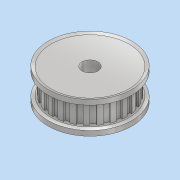
# Autodesk Inventor part: Koło zębate 21 T5 24 2F
Saved by Autodesk Inventor 2018 (Build 220112000, 112)
## iProperties
Created: 2019-01-23
Part Number: Koło zębate 21 T5 24 2F
Material: Ogólny
Document SubType Name: Modeling
Designer: Dawid
Density: 1 g/cm^3
Appearance: Aluminium — ciemne
Author: Dawid
Autodesk Inventor part; units mm, degrees
ref_plane "YZ Plane" through (0, 0, 0) normal (1, 0, 0) x (0, 1, 0)
ref_plane "XZ Plane" through (0, 0, 0) normal (0, 1, 0) x (-1, 0, 0)
ref_plane "XY Plane" through (0, 0, 0) normal (0, 0, 1) x (1, 0, 0)
sketch "Szkic1" plane through (0, 0, 0) normal (0, 0, 1) x (1, 0, 0)
  arc A0 (2.4408, 18.54) -> (0, 18.7) centre (0, 0) ccw
  arc A1 (0, 17.7) -> (2.3103, 17.5486) centre (0, 0) ccw
  line L0 (0, 0) -> (0, 18.7)
  line L1 (0, 0) -> (2.4408, 18.54)
  line L2 (0, 0) -> (18.7, 0) construction
  dimension "d0" = 37.4
  dimension "d1" = 35.4
  dimension "d2" = 82.5
  constraints: 6 end point, 4 point on circle, 2 centre point, 2 coincident, 2 point on line, 1 equal length, 1 horizontal, 1 vertical
  measures "d0" diameter of A0
  measures "d1" diameter of A1
  measures "d2" angle of L2 L1
extrude "Wyciągnięcie proste1" add sketch "Szkic1" along normal blind 21
pattern_circular "Szyk kołowy1" count 24 over 360 about axis through (0, 0, 0) along (0, 0, 1) of "Wyciągnięcie proste1"
sketch "Szkic2" plane through (0, 0, 0) normal (0, 0, -1) x (-1, 0, 0)
  line L0 (0, 18.7) -> (0, 17.7) projected
  arc A0 (0, 18.7) -> (-2.4408, 18.54) centre (0, 0) ccw projected
  line L1 (-2.3103, 17.5486) -> (-2.4408, 18.54) projected
  arc A1 (-2.3103, 17.5486) -> (-4.5811, 17.0969) centre (0, 0) ccw projected
  line L2 (-4.8399, 18.0628) -> (-4.5811, 17.0969) projected
  arc A2 (-4.8399, 18.0628) -> (-7.1562, 17.2765) centre (0, 0) ccw projected
  line L3 (-6.7735, 16.3527) -> (-7.1562, 17.2765) projected
  arc A3 (-6.7735, 16.3527) -> (-8.85, 15.3286) centre (0, 0) ccw projected
  line L4 (-9.35, 16.1947) -> (-8.85, 15.3286) projected
  arc A4 (-9.35, 16.1947) -> (-11.3838, 14.8357) centre (0, 0) ccw projected
  line L5 (-10.7751, 14.0424) -> (-11.3838, 14.8357) projected
  arc A5 (-10.7751, 14.0424) -> (-12.5158, 12.5158) centre (0, 0) ccw projected
  line L6 (-13.2229, 13.2229) -> (-12.5158, 12.5158) projected
  arc A6 (-13.2229, 13.2229) -> (-14.8357, 11.3838) centre (0, 0) ccw projected
  line L7 (-14.0424, 10.7751) -> (-14.8357, 11.3838) projected
  arc A7 (-14.0424, 10.7751) -> (-15.3286, 8.85) centre (0, 0) ccw projected
  line L8 (-16.1947, 9.35) -> (-15.3286, 8.85) projected
  arc A8 (-16.1947, 9.35) -> (-17.2765, 7.1562) centre (0, 0) ccw projected
  line L9 (-16.3527, 6.7735) -> (-17.2765, 7.1562) projected
  arc A9 (-16.3527, 6.7735) -> (-17.0969, 4.5811) centre (0, 0) ccw projected
  line L10 (-18.0628, 4.8399) -> (-17.0969, 4.5811) projected
  arc A10 (-18.0628, 4.8399) -> (-18.54, 2.4408) centre (0, 0) ccw projected
  line L11 (-17.5486, 2.3103) -> (-18.54, 2.4408) projected
  arc A11 (-17.5486, 2.3103) -> (-17.7, 0) centre (0, 0) ccw projected
  line L12 (-18.7, 0) -> (-17.7, 0) projected
  arc A12 (-18.7, 0) -> (-18.54, -2.4408) centre (0, 0) ccw projected
  line L13 (-17.5486, -2.3103) -> (-18.54, -2.4408) projected
  arc A13 (-17.5486, -2.3103) -> (-17.0969, -4.5811) centre (0, 0) ccw projected
  line L14 (-18.0628, -4.8399) -> (-17.0969, -4.5811) projected
  arc A14 (-18.0628, -4.8399) -> (-17.2765, -7.1562) centre (0, 0) ccw projected
  line L15 (-16.3527, -6.7735) -> (-17.2765, -7.1562) projected
  arc A15 (-16.3527, -6.7735) -> (-15.3286, -8.85) centre (0, 0) ccw projected
  line L16 (-16.1947, -9.35) -> (-15.3286, -8.85) projected
  arc A16 (-16.1947, -9.35) -> (-14.8357, -11.3838) centre (0, 0) ccw projected
  line L17 (-14.0424, -10.7751) -> (-14.8357, -11.3838) projected
  arc A17 (-14.0424, -10.7751) -> (-12.5158, -12.5158) centre (0, 0) ccw projected
  line L18 (-13.2229, -13.2229) -> (-12.5158, -12.5158) projected
  arc A18 (-13.2229, -13.2229) -> (-11.3838, -14.8357) centre (0, 0) ccw projected
  line L19 (-10.7751, -14.0424) -> (-11.3838, -14.8357) projected
  arc A19 (-10.7751, -14.0424) -> (-8.85, -15.3286) centre (0, 0) ccw projected
  line L20 (-9.35, -16.1947) -> (-8.85, -15.3286) projected
  arc A20 (-9.35, -16.1947) -> (-7.1562, -17.2765) centre (0, 0) ccw projected
  line L21 (-6.7735, -16.3527) -> (-7.1562, -17.2765) projected
  arc A21 (-6.7735, -16.3527) -> (-4.5811, -17.0969) centre (0, 0) ccw projected
  line L22 (-4.8399, -18.0628) -> (-4.5811, -17.0969) projected
  arc A22 (-4.8399, -18.0628) -> (-2.4408, -18.54) centre (0, 0) ccw projected
  line L23 (-2.3103, -17.5486) -> (-2.4408, -18.54) projected
  arc A23 (-2.3103, -17.5486) -> (0, -17.7) centre (0, 0) ccw projected
  line L24 (0, -18.7) -> (0, -17.7) projected
  arc A24 (0, -18.7) -> (2.4408, -18.54) centre (0, 0) ccw projected
  line L25 (2.3103, -17.5486) -> (2.4408, -18.54) projected
  arc A25 (2.3103, -17.5486) -> (4.5811, -17.0969) centre (0, 0) ccw projected
  line L26 (4.8399, -18.0628) -> (4.5811, -17.0969) projected
  arc A26 (4.8399, -18.0628) -> (7.1562, -17.2765) centre (0, 0) ccw projected
  line L27 (6.7735, -16.3527) -> (7.1562, -17.2765) projected
  arc A27 (6.7735, -16.3527) -> (8.85, -15.3286) centre (0, 0) ccw projected
  line L28 (9.35, -16.1947) -> (8.85, -15.3286) projected
  arc A28 (9.35, -16.1947) -> (11.3838, -14.8357) centre (0, 0) ccw projected
  line L29 (10.7751, -14.0424) -> (11.3838, -14.8357) projected
  arc A29 (10.7751, -14.0424) -> (12.5158, -12.5158) centre (0, 0) ccw projected
  line L30 (13.2229, -13.2229) -> (12.5158, -12.5158) projected
  arc A30 (13.2229, -13.2229) -> (14.8357, -11.3838) centre (0, 0) ccw projected
  line L31 (14.0424, -10.7751) -> (14.8357, -11.3838) projected
  arc A31 (14.0424, -10.7751) -> (15.3286, -8.85) centre (0, 0) ccw projected
  line L32 (16.1947, -9.35) -> (15.3286, -8.85) projected
  arc A32 (16.1947, -9.35) -> (17.2765, -7.1562) centre (0, 0) ccw projected
  line L33 (16.3527, -6.7735) -> (17.2765, -7.1562) projected
  arc A33 (16.3527, -6.7735) -> (17.0969, -4.5811) centre (0, 0) ccw projected
  line L34 (18.0628, -4.8399) -> (17.0969, -4.5811) projected
  arc A34 (18.0628, -4.8399) -> (18.54, -2.4408) centre (0, 0) ccw projected
  line L35 (17.5486, -2.3103) -> (18.54, -2.4408) projected
  arc A35 (17.5486, -2.3103) -> (17.7, 0) centre (0, 0) ccw projected
  line L36 (18.7, 0) -> (17.7, 0) projected
  arc A36 (18.7, 0) -> (18.54, 2.4408) centre (0, 0) ccw projected
  line L37 (17.5486, 2.3103) -> (18.54, 2.4408) projected
  arc A37 (17.5486, 2.3103) -> (17.0969, 4.5811) centre (0, 0) ccw projected
  line L38 (18.0628, 4.8399) -> (17.0969, 4.5811) projected
  arc A38 (18.0628, 4.8399) -> (17.2765, 7.1562) centre (0, 0) ccw projected
  line L39 (16.3527, 6.7735) -> (17.2765, 7.1562) projected
  arc A39 (16.3527, 6.7735) -> (15.3286, 8.85) centre (0, 0) ccw projected
  line L40 (16.1947, 9.35) -> (15.3286, 8.85) projected
  arc A40 (16.1947, 9.35) -> (14.8357, 11.3838) centre (0, 0) ccw projected
  line L41 (14.0424, 10.7751) -> (14.8357, 11.3838) projected
  arc A41 (14.0424, 10.7751) -> (12.5158, 12.5158) centre (0, 0) ccw projected
  line L42 (13.2229, 13.2229) -> (12.5158, 12.5158) projected
  arc A42 (13.2229, 13.2229) -> (11.3838, 14.8357) centre (0, 0) ccw projected
  line L43 (10.7751, 14.0424) -> (11.3838, 14.8357) projected
  arc A43 (10.7751, 14.0424) -> (8.85, 15.3286) centre (0, 0) ccw projected
  line L44 (9.35, 16.1947) -> (8.85, 15.3286) projected
  arc A44 (9.35, 16.1947) -> (7.1562, 17.2765) centre (0, 0) ccw projected
  line L45 (6.7735, 16.3527) -> (7.1562, 17.2765) projected
  arc A45 (6.7735, 16.3527) -> (4.5811, 17.0969) centre (0, 0) ccw projected
  line L46 (4.8399, 18.0628) -> (4.5811, 17.0969) projected
  arc A46 (4.8399, 18.0628) -> (2.4408, 18.54) centre (0, 0) ccw projected
  line L47 (2.3103, 17.5486) -> (2.4408, 18.54) projected
  arc A47 (2.3103, 17.5486) -> (0, 17.7) centre (0, 0) ccw projected
  circle A48 centre (0, 0) radius 12
  dimension "d8" = 24
  constraints: 1 centre point, 1 coincident
  measures "d8" diameter of A48
extrude "Wyciągnięcie proste2" cut sketch "Szkic2" against normal blind 6
sketch "Szkic3" plane through (0, 0, 0) normal (1, 0, 0) x (0, 1, 0)
  line L0 (0, 6) -> (-2.3103, 6) projected
  line L1 (0, 6) -> (19.5, 6)
  line L2 (21, 6) -> (21, 5.5)
  line L3 (19.5, 6) -> (21, 5.5)
  line L4 (21, 8) -> (19.5, 8.5)
  line L5 (21, 6) -> (21, 8)
  line L6 (0, 6) -> (0, 8.5)
  line L7 (0, 6) -> (0, 21)
  line L8 (0, 8.5) -> (19.5, 8.5)
  line L9 (0, 21) -> (-2.3103, 21) projected
  line L10 (0, 21) -> (19.5, 21)
  line L11 (21, 21) -> (21, 21.5)
  line L12 (19.5, 21) -> (21, 21.5)
  line L13 (21, 21) -> (21, 19)
  line L14 (19.5, 18.5) -> (0, 18.5)
  line L15 (19.5, 18.5) -> (21, 19)
  point P0 (0, 0)
  dimension "d16" = 2.5
  constraints: 28 end point, 2 point on line
  measures "d16" distance of L0.start L6.end
revolve "Obrót1" add sketch "Szkic3" angle 360 about axis through (0, 0, 6) along (0, 0, 1)
sketch "Szkic4" plane through (0, 0, 0) normal (0, 0, -1) x (-1, 0, 0)
  circle A0 centre (0, 0) radius 4
  dimension "d24" = 8
  constraints: 1 centre point, 1 coincident
  measures "d24" diameter of A0
extrude "Wyciągnięcie proste3" cut sketch "Szkic4" against normal up to next
